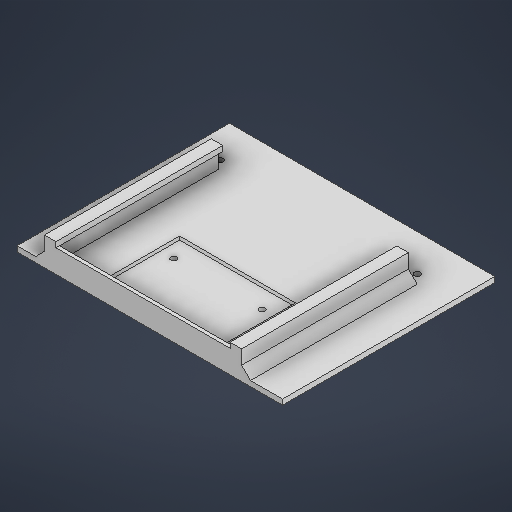
# Autodesk Inventor part: TOPLeft
Saved by Autodesk Inventor 2026.1 (Build 301233020, 233B)
## iProperties
Created: 2026-07-07
Part Number: TOPLeft
Material: Generic
Document SubType Name: Modeling
Designer: pleased
Density: 1 g/cm^3
Appearance: Default
Author: pleased
Autodesk Inventor part; units mm, degrees
ref_plane "YZ Plane" through (0, 0, 0) normal (1, 0, 0) x (0, 1, 0)
ref_plane "XZ Plane" through (0, 0, 0) normal (0, 1, 0) x (-1, 0, 0)
ref_plane "XY Plane" through (0, 0, 0) normal (0, 0, 1) x (1, 0, 0)
sketch "Sketch1" plane through (0, 0, 0) normal (0, 1, 0) x (-1, 0, 0)
  line L0 (0, 80) -> (150, 80)
  line L1 (150, 80) -> (150, 0)
  line L2 (150, 0) -> (0, 0)
  line L3 (0, 0) -> (0, 80)
  point P0 (0, 0)
  dimension "d0" = 150
  dimension "d1" = 80
  constraints: 8 end point, 2 parallel, 1 horizontal, 1 perpendicular
  measures "d0" distance of L1.end L2.end
  measures "d1" distance of L0.end L1.end
extrude "Extrusion1" add sketch "Sketch1" along normal blind 3
sketch "Sketch2" plane through (0, 3, 0) normal (0, 1, 0) x (1, 0, 0)
  circle A0 centre (-100.5, -71) radius 1.65
  circle A1 centre (-100.5, -41) radius 1.65
  circle A2 centre (-50.5, -71) radius 1.65
  circle A3 centre (-50.5, -41) radius 1.65
  point P0 (0, 0)
  point P1 (-93.7, -18)
  point P2 (-92, -41)
  point P3 (-92, -71)
  point P4 (-58, -18)
  dimension "d5" = 3.3
  dimension "d6" = 3.3
  dimension "d7" = 3.3
  dimension "d8" = 3.3
  constraints: 4 centre point, 4 coincident
  measures "d5" diameter of A0
  measures "d6" diameter of A1
  measures "d7" diameter of A2
  measures "d8" diameter of A3
extrude "Extrusion2" cut sketch "Sketch2" against normal blind 3
sketch "Sketch3" plane through (0, 3, 0) normal (0, 1, 0) x (1, 0, 0)
  line L0 (-107.9014, -77.0296) -> (-44.3595, -77.0296)
  line L1 (-44.3595, -77.0296) -> (-44.3595, -30.3031)
  line L2 (-44.3595, -30.3031) -> (-107.9014, -30.3031)
  line L3 (-107.9014, -30.3031) -> (-107.9014, -77.0296)
  point P0 (0, 0)
  constraints: 8 end point, 2 parallel, 1 horizontal, 1 perpendicular
extrude "Extrusion3" cut sketch "Sketch3" against normal blind 1
chamfer "Chamfer1" distance 1 angle 45 4 edges at (-107.9014, 3, 53.6663) (-76.1304, 3, 30.3031) (-44.3595, 3, 53.6663) (-76.1304, 3, 77.0296)
sketch "Sketch4" plane through (0, 3, 0) normal (0, 1, 0) x (1, 0, 0)
  line L0 (-27.118, 12.3565) -> (-130.518, 12.3565)
  line L1 (-130.518, 12.3565) -> (-130.518, -78.0435)
  line L2 (-130.518, -78.0435) -> (-27.118, -78.0435)
  line L3 (-27.118, -78.0435) -> (-27.118, 12.3565)
  line L4 (-27.118, -78.0435) -> (-23.118, -78.0435)
  line L5 (-23.118, -78.0435) -> (-23.118, 14.2127)
  line L6 (-23.118, 14.2127) -> (-27.118, 14.2127)
  line L7 (-27.118, 14.2127) -> (-27.118, -78.0435)
  line L8 (-130.518, -78.0435) -> (-134.518, -78.0435)
  line L9 (-134.518, -78.0435) -> (-134.518, 14.2127)
  line L10 (-134.518, 14.2127) -> (-130.518, 14.2127)
  line L11 (-130.518, 14.2127) -> (-130.518, -78.0435)
  line L12 (-150, -80) -> (0, -80) projected
  line L13 (-134.518, -78.0435) -> (-23.118, -78.0435)
  line L14 (-23.118, -78.0435) -> (-23.118, -80)
  line L15 (-23.118, -80) -> (-134.518, -80)
  line L16 (-134.518, -80) -> (-134.518, -78.0435)
  point P0 (0, 0)
  dimension "d16" = 103.4
  dimension "d17" = 90.4
  dimension "d21" = 4
  dimension "d22" = 4
  constraints: 32 end point, 8 parallel, 4 horizontal, 4 perpendicular, 3 point on line
  measures "d16" distance of L2.end L1.end
  measures "d17" distance of L1.end L0.end
  measures "d21" distance of L6.end L5.end
  measures "d22" distance of L9.end L10.end
move faces "Move1" translate (0, 0, -40) faces at (-50, 1, 0)
extrude "Extrusion4" add sketch "Sketch4" along normal blind 10 contours L7 L6 L5 L4 L3 | L1 L8 L9 L10 L11 | L4 L14 L12 L16 L8 L2
sketch "Sketch5" plane through (0, 13, 0) normal (0, 1, 0) x (1, 0, 0)
  line L0 (-23.118, 14.2127) -> (-23.118, -80) projected
  line L1 (-134.518, -80) -> (-23.118, -80) projected
  line L2 (-23.118, 14.2127) -> (-29.618, 14.2127)
  line L3 (-29.618, 14.2127) -> (-29.618, -80)
  line L4 (-29.618, -80) -> (-23.118, -80)
  line L5 (-23.118, -80) -> (-23.118, 14.2127)
  line L6 (-134.518, 14.2127) -> (-128.018, 14.2127)
  line L7 (-128.018, 14.2127) -> (-128.018, -80)
  line L8 (-128.018, -80) -> (-134.518, -80)
  line L9 (-134.518, -80) -> (-134.518, 14.2127)
  point P0 (0, 0)
  point P1 (-27.118, 14.2127)
  point P2 (-27.118, -78.0435)
  point P3 (-130.518, 14.2127)
  point P4 (-130.518, -78.0435)
  dimension "d25" = 6.5
  dimension "d26" = 6.5
  constraints: 16 end point, 4 parallel, 2 horizontal, 2 perpendicular, 2 point on line
  measures "d25" distance of L4.end L3.end
  measures "d26" distance of L7.end L8.end
extrude "Extrusion5" add sketch "Sketch5" along normal blind 3
sketch "Sketch6" plane through (0, 3, 0) normal (0, 1, 0) x (1, 0, 0)
  line L0 (-27.118, 14.2127) -> (-23.118, 14.2127) projected
  line L1 (-23.118, 14.2127) -> (-134.518, 14.2127)
  line L2 (-134.518, 14.2127) -> (-134.518, 19.2127)
  line L3 (-134.518, 19.2127) -> (-23.118, 19.2127)
  line L4 (-23.118, 19.2127) -> (-23.118, 14.2127)
  circle A0 centre (-134.518, 19.2127) radius 1.75
  circle A1 centre (-23.118, 19.2127) radius 1.75
  point P0 (0, 0)
  dimension "d29" = 5
  dimension "d30" = 3.5
  dimension "d31" = 3.5
  constraints: 8 end point, 2 centre point, 2 coincident, 2 parallel, 1 horizontal, 1 perpendicular
  measures "d29" distance of L1.end L2.end
  measures "d30" diameter of A0
  measures "d31" diameter of A1
extrude "Extrusion6" cut sketch "Sketch6" against normal blind 3 contours A1 L3 L4 | L4 L3 A1 | A0 L3 L2 | L2 L3 A0
sketch "Sketch7" plane through (0, 0, 0) normal (0, -1, 0) x (1, 0, 0)
  line L0 (-26.618, -22.7127) -> (-19.618, -22.7127)
  line L1 (-19.618, -22.7127) -> (-19.618, -15.7127)
  line L2 (-19.618, -15.7127) -> (-26.618, -15.7127)
  line L3 (-26.618, -15.7127) -> (-26.618, -22.7127)
  circle A0 centre (-23.118, -19.2127) radius 1.75 projected
  line L4 (-26.618, -22.7127) -> (-19.618, -15.7127) construction
  line L5 (-19.618, -22.7127) -> (-26.618, -15.7127) construction
  line L6 (-138.018, -22.7127) -> (-131.018, -22.7127)
  line L7 (-131.018, -22.7127) -> (-131.018, -15.7127)
  line L8 (-131.018, -15.7127) -> (-138.018, -15.7127)
  line L9 (-138.018, -15.7127) -> (-138.018, -22.7127)
  circle A1 centre (-134.518, -19.2127) radius 1.75 projected
  line L10 (-138.018, -22.7127) -> (-131.018, -15.7127) construction
  line L11 (-131.018, -22.7127) -> (-138.018, -15.7127) construction
  point P0 (0, 0)
  dimension "d34" = 7
  dimension "d35" = 7
  dimension "d36" = 7
  dimension "d37" = 7
  constraints: 24 end point, 4 midpoint, 4 parallel, 2 horizontal, 2 perpendicular
  measures "d34" distance of L2.end L1.end
  measures "d35" distance of L1.end L0.end
  measures "d36" distance of L8.end L7.end
  measures "d37" distance of L7.end L6.end
extrude "Extrusion7" add sketch "Sketch7" along normal blind 5 contours L3 L2 L1 L0 | A0 | L9 L8 L7 L6 | A1
move faces "Move2" translate (0, -1, 0) faces at (-23.1883, 0, -18.7009) (-133.6676, 0, -18.8259)
chamfer "Chamfer2" distance 5 angle 45 8 edges at (-134.518, 0, -15.7127) (-138.018, 0, -19.2127) (-134.518, 0, -22.7127) (-131.018, 0, -19.2127) (-23.118, 0, -22.7127) (-26.618, 0, -19.2127) (-23.118, 0, -15.7127) (-19.618, 0, -19.2127)
chamfer "Chamfer3" distance 5 angle 45 2 edges at (-134.518, 3, 32.8937) (-23.118, 3, 32.8937)
body "Solid1"
